Autodesk Inventor part; units mm, degrees
(part 2 of 2)
  spline S162 degree 2 poles (-0.0394, -200.6231) (-0.0431, -200.6898) (-0.0505, -200.8158) (-0.0505, -200.9121) knots 0 0 0 1 2 2 2
  spline S163 degree 2 poles (-0.0505, -200.9121) (-0.0505, -201.3864) (0.1348, -201.9681) (0.2755, -202.12) knots 0 0 0 1 2 2 2
  spline S164 degree 2 poles (0.2755, -202.12) (0.4052, -202.2645) (0.6868, -202.3793) (0.8461, -202.3793) knots 0 0 0 1 2 2 2
  spline S165 degree 2 poles (0.8461, -202.3793) (1.2166, -202.3793) (1.6723, -201.8532) (1.6723, -201.3271) knots 0 0 0 1 2 2 2
  line L137 (4.7364, -198.0074) -> (2.9469, -203.7761)
  line L138 (2.9469, -203.7761) -> (2.4282, -203.7761)
  line L139 (2.4282, -203.7761) -> (4.2103, -198.0074)
  line L140 (4.2103, -198.0074) -> (4.7364, -198.0074)
  line L141 (8.0598, -202.7832) -> (5.2403, -202.7832)
  line L142 (5.2403, -202.7832) -> (5.2403, -202.1348)
  spline S166 degree 2 poles (5.2403, -202.1348) (5.5441, -201.8495) (6.085, -201.3197) (6.3444, -201.0344) knots 0 0 0 1 2 2 2
  spline S167 degree 2 poles (6.3444, -201.0344) (6.8668, -200.4601) (7.2484, -199.771) (7.2484, -199.4042) knots 0 0 0 1 2 2 2
  spline S168 degree 2 poles (7.2484, -199.4042) (7.2484, -199.2115) (7.1298, -198.9225) (7.0224, -198.8299) knots 0 0 0 1 2 2 2
  spline S169 degree 2 poles (7.0224, -198.8299) (6.9149, -198.7373) (6.6334, -198.6447) (6.4629, -198.6447) knots 0 0 0 1 2 2 2
  spline S170 degree 2 poles (6.4629, -198.6447) (6.2999, -198.6447) (5.9665, -198.7262) (5.8146, -198.7892) knots 0 0 0 1 2 2 2
  spline S171 degree 2 poles (5.8146, -198.7892) (5.6849, -198.841) (5.4441, -198.9892) (5.37, -199.0411) knots 0 0 0 1 2 2 2
  line L143 (5.37, -199.0411) -> (5.3366, -199.0411)
  line L144 (5.3366, -199.0411) -> (5.3366, -198.389)
  spline S172 degree 2 poles (5.3366, -198.389) (5.5256, -198.2964) (6.2036, -198.1148) (6.5074, -198.1148) knots 0 0 0 1 2 2 2
  spline S173 degree 2 poles (6.5074, -198.1148) (7.1484, -198.1148) (7.8708, -198.7929) (7.8708, -199.3708) knots 0 0 0 1 2 2 2
  spline S174 degree 2 poles (7.8708, -199.3708) (7.8708, -199.6413) (7.7449, -200.0933) (7.6337, -200.286) knots 0 0 0 1 2 2 2
  spline S175 degree 2 poles (7.6337, -200.286) (7.5226, -200.4861) (7.2002, -200.8788) (7.0224, -201.0677) knots 0 0 0 1 2 2 2
  spline S176 degree 2 poles (7.0224, -201.0677) (6.7334, -201.3827) (6.0257, -202.057) (5.8146, -202.2534) knots 0 0 0 1 2 2 2
  line L145 (5.8146, -202.2534) -> (8.0598, -202.2534)
  line L146 (8.0598, -202.2534) -> (8.0598, -202.7832)
  spline S177 degree 2 poles (10.0531, -202.8869) (9.7122, -202.8869) (9.1528, -202.6831) (8.9564, -202.4942) knots 0 0 0 1 2 2 2
  spline S178 degree 2 poles (8.9564, -202.4942) (8.7638, -202.3089) (8.5637, -201.805) (8.5637, -201.5198) knots 0 0 0 1 2 2 2
  spline S179 degree 2 poles (8.5637, -201.5198) (8.5637, -201.1493) (8.9601, -200.5268) (9.338, -200.3416) knots 0 0 0 1 2 2 2
  line L147 (9.338, -200.3416) -> (9.338, -200.323)
  spline S180 degree 2 poles (9.338, -200.323) (9.0009, -200.1267) (8.6748, -199.6598) (8.6748, -199.3116) knots 0 0 0 1 2 2 2
  spline S181 degree 2 poles (8.6748, -199.3116) (8.6748, -198.7966) (9.4529, -198.1074) (10.0531, -198.1074) knots 0 0 0 1 2 2 2
  spline S182 degree 2 poles (10.0531, -198.1074) (10.6755, -198.1074) (11.4277, -198.7595) (11.4277, -199.2708) knots 0 0 0 1 2 2 2
  spline S183 degree 2 poles (11.4277, -199.2708) (11.4277, -199.5783) (11.0683, -200.1785) (10.7311, -200.349) knots 0 0 0 1 2 2 2
  line L148 (10.7311, -200.349) -> (10.7311, -200.3675)
  spline S184 degree 2 poles (10.7311, -200.3675) (11.1313, -200.5528) (11.5425, -201.0863) (11.5425, -201.5086) knots 0 0 0 1 2 2 2
  spline S185 degree 2 poles (11.5425, -201.5086) (11.5425, -202.094) (10.6904, -202.8869) (10.0531, -202.8869) knots 0 0 0 1 2 2 2
  spline S186 degree 2 poles (10.9127, -201.5679) (10.9127, -201.2863) (10.6904, -200.9529) (10.3754, -200.7825) knots 0 0 0 1 2 2 2
  spline S187 degree 2 poles (10.3754, -200.7825) (10.2717, -200.7232) (9.9234, -200.5861) (9.7048, -200.4972) knots 0 0 0 1 2 2 2
  spline S188 degree 2 poles (9.7048, -200.4972) (9.4529, -200.6639) (9.1824, -201.1604) (9.1824, -201.4753) knots 0 0 0 1 2 2 2
  spline S189 degree 2 poles (9.1824, -201.4753) (9.1824, -201.8903) (9.6826, -202.4312) (10.0605, -202.4312) knots 0 0 0 1 2 2 2
  spline S190 degree 2 poles (10.0605, -202.4312) (10.4458, -202.4312) (10.9127, -201.9681) (10.9127, -201.5679) knots 0 0 0 1 2 2 2
  spline S191 degree 2 poles (10.8275, -199.2782) (10.8275, -198.9707) (10.4162, -198.5594) (10.0494, -198.5594) knots 0 0 0 1 2 2 2
  spline S192 degree 2 poles (10.0494, -198.5594) (9.7159, -198.5594) (9.2899, -198.9262) (9.2899, -199.2412) knots 0 0 0 1 2 2 2
  spline S193 degree 2 poles (9.2899, -199.2412) (9.2899, -199.4672) (9.5085, -199.7821) (9.7271, -199.9081) knots 0 0 0 1 2 2 2
  spline S194 degree 2 poles (9.7271, -199.9081) (9.8197, -199.9599) (10.2124, -200.1415) (10.3717, -200.1934) knots 0 0 0 1 2 2 2
  spline S195 degree 2 poles (10.3717, -200.1934) (10.6385, -199.9896) (10.8275, -199.5561) (10.8275, -199.2782) knots 0 0 0 1 2 2 2
  line L149 (14.0027, -198.0074) -> (12.2131, -203.7761)
  line L150 (12.2131, -203.7761) -> (11.6944, -203.7761)
  line L151 (11.6944, -203.7761) -> (13.4765, -198.0074)
  line L152 (13.4765, -198.0074) -> (14.0027, -198.0074)
  line L153 (17.3261, -202.7832) -> (14.5065, -202.7832)
  line L154 (14.5065, -202.7832) -> (14.5065, -202.1348)
  spline S196 degree 2 poles (14.5065, -202.1348) (14.8104, -201.8495) (15.3513, -201.3197) (15.6106, -201.0344) knots 0 0 0 1 2 2 2
  spline S197 degree 2 poles (15.6106, -201.0344) (16.133, -200.4601) (16.5147, -199.771) (16.5147, -199.4042) knots 0 0 0 1 2 2 2
  spline S198 degree 2 poles (16.5147, -199.4042) (16.5147, -199.2115) (16.3961, -198.9225) (16.2887, -198.8299) knots 0 0 0 1 2 2 2
  spline S199 degree 2 poles (16.2887, -198.8299) (16.1812, -198.7373) (15.8996, -198.6447) (15.7292, -198.6447) knots 0 0 0 1 2 2 2
  spline S200 degree 2 poles (15.7292, -198.6447) (15.5662, -198.6447) (15.2327, -198.7262) (15.0808, -198.7892) knots 0 0 0 1 2 2 2
  spline S201 degree 2 poles (15.0808, -198.7892) (14.9511, -198.841) (14.7103, -198.9892) (14.6362, -199.0411) knots 0 0 0 1 2 2 2
  line L155 (14.6362, -199.0411) -> (14.6029, -199.0411)
  line L156 (14.6029, -199.0411) -> (14.6029, -198.389)
  spline S202 degree 2 poles (14.6029, -198.389) (14.7918, -198.2964) (15.4698, -198.1148) (15.7737, -198.1148) knots 0 0 0 1 2 2 2
  spline S203 degree 2 poles (15.7737, -198.1148) (16.4146, -198.1148) (17.1371, -198.7929) (17.1371, -199.3708) knots 0 0 0 1 2 2 2
  spline S204 degree 2 poles (17.1371, -199.3708) (17.1371, -199.6413) (17.0111, -200.0933) (16.9, -200.286) knots 0 0 0 1 2 2 2
  spline S205 degree 2 poles (16.9, -200.286) (16.7888, -200.4861) (16.4665, -200.8788) (16.2887, -201.0677) knots 0 0 0 1 2 2 2
  spline S206 degree 2 poles (16.2887, -201.0677) (15.9997, -201.3827) (15.292, -202.057) (15.0808, -202.2534) knots 0 0 0 1 2 2 2
  line L157 (15.0808, -202.2534) -> (17.3261, -202.2534)
  line L158 (17.3261, -202.2534) -> (17.3261, -202.7832)
  spline S207 degree 2 poles (20.7829, -200.4972) (20.7829, -201.7272) (20.0678, -202.8795) (19.3231, -202.8795) knots 0 0 0 1 2 2 2
  spline S208 degree 2 poles (19.3231, -202.8795) (18.5672, -202.8795) (17.8596, -201.705) (17.8596, -200.5009) knots 0 0 0 1 2 2 2
  spline S209 degree 2 poles (17.8596, -200.5009) (17.8596, -199.2634) (18.5747, -198.1185) (19.3231, -198.1185) knots 0 0 0 1 2 2 2
  spline S210 degree 2 poles (19.3231, -198.1185) (20.0752, -198.1185) (20.7829, -199.3042) (20.7829, -200.4972) knots 0 0 0 1 2 2 2
  spline S211 degree 2 poles (19.9974, -201.8903) (20.0863, -201.6643) (20.1604, -200.9677) (20.1604, -200.4972) knots 0 0 0 1 2 2 2
  spline S212 degree 2 poles (20.1604, -200.4972) (20.1604, -200.0266) (20.0863, -199.3338) (19.9937, -199.1004) knots 0 0 0 1 2 2 2
  spline S213 degree 2 poles (19.9937, -199.1004) (19.9011, -198.867) (19.5787, -198.6261) (19.3231, -198.6261) knots 0 0 0 1 2 2 2
  spline S214 degree 2 poles (19.3231, -198.6261) (19.0674, -198.6261) (18.7377, -198.867) (18.6413, -199.1078) knots 0 0 0 1 2 2 2
  spline S215 degree 2 poles (18.6413, -199.1078) (18.5487, -199.3412) (18.482, -200.0526) (18.482, -200.5009) knots 0 0 0 1 2 2 2
  spline S216 degree 2 poles (18.482, -200.5009) (18.482, -200.9825) (18.5413, -201.6272) (18.6376, -201.8791) knots 0 0 0 1 2 2 2
  spline S217 degree 2 poles (18.6376, -201.8791) (18.7266, -202.1163) (19.0563, -202.3719) (19.3231, -202.3719) knots 0 0 0 1 2 2 2
  spline S218 degree 2 poles (19.3231, -202.3719) (19.575, -202.3719) (19.9048, -202.1311) (19.9974, -201.8903) knots 0 0 0 1 2 2 2
  line L159 (24.1878, -202.7832) -> (21.3682, -202.7832)
  line L160 (21.3682, -202.7832) -> (21.3682, -202.1348)
  spline S219 degree 2 poles (21.3682, -202.1348) (21.6721, -201.8495) (22.213, -201.3197) (22.4723, -201.0344) knots 0 0 0 1 2 2 2
  spline S220 degree 2 poles (22.4723, -201.0344) (22.9948, -200.4601) (23.3764, -199.771) (23.3764, -199.4042) knots 0 0 0 1 2 2 2
  spline S221 degree 2 poles (23.3764, -199.4042) (23.3764, -199.2115) (23.2578, -198.9225) (23.1504, -198.8299) knots 0 0 0 1 2 2 2
  spline S222 degree 2 poles (23.1504, -198.8299) (23.0429, -198.7373) (22.7613, -198.6447) (22.5909, -198.6447) knots 0 0 0 1 2 2 2
  spline S223 degree 2 poles (22.5909, -198.6447) (22.4279, -198.6447) (22.0944, -198.7262) (21.9425, -198.7892) knots 0 0 0 1 2 2 2
  spline S224 degree 2 poles (21.9425, -198.7892) (21.8128, -198.841) (21.572, -198.9892) (21.4979, -199.0411) knots 0 0 0 1 2 2 2
  line L161 (21.4979, -199.0411) -> (21.4646, -199.0411)
  line L162 (21.4646, -199.0411) -> (21.4646, -198.389)
  spline S225 degree 2 poles (21.4646, -198.389) (21.6535, -198.2964) (22.3316, -198.1148) (22.6354, -198.1148) knots 0 0 0 1 2 2 2
  spline S226 degree 2 poles (22.6354, -198.1148) (23.2763, -198.1148) (23.9988, -198.7929) (23.9988, -199.3708) knots 0 0 0 1 2 2 2
  spline S227 degree 2 poles (23.9988, -199.3708) (23.9988, -199.6413) (23.8728, -200.0933) (23.7617, -200.286) knots 0 0 0 1 2 2 2
  spline S228 degree 2 poles (23.7617, -200.286) (23.6505, -200.4861) (23.3282, -200.8788) (23.1504, -201.0677) knots 0 0 0 1 2 2 2
  spline S229 degree 2 poles (23.1504, -201.0677) (22.8614, -201.3827) (22.1537, -202.057) (21.9425, -202.2534) knots 0 0 0 1 2 2 2
  line L163 (21.9425, -202.2534) -> (24.1878, -202.2534)
  line L164 (24.1878, -202.2534) -> (24.1878, -202.7832)
  spline S230 degree 2 poles (27.689, -201.3012) (27.689, -201.6531) (27.4556, -202.2497) (27.2592, -202.4497) knots 0 0 0 1 2 2 2
  spline S231 degree 2 poles (27.2592, -202.4497) (27.0555, -202.6609) (26.5442, -202.8795) (26.2366, -202.8795) knots 0 0 0 1 2 2 2
  spline S232 degree 2 poles (26.2366, -202.8795) (25.9291, -202.8795) (25.4215, -202.672) (25.2289, -202.4645) knots 0 0 0 1 2 2 2
  spline S233 degree 2 poles (25.2289, -202.4645) (24.9918, -202.2163) (24.725, -201.3827) (24.725, -200.7751) knots 0 0 0 1 2 2 2
  spline S234 degree 2 poles (24.725, -200.7751) (24.725, -200.1785) (24.9695, -199.2189) (25.2252, -198.8633) knots 0 0 0 1 2 2 2
  spline S235 degree 2 poles (25.2252, -198.8633) (25.4734, -198.515) (26.2589, -198.126) (26.7739, -198.126) knots 0 0 0 1 2 2 2
  spline S236 degree 2 poles (26.7739, -198.126) (26.9258, -198.126) (27.1925, -198.1556) (27.2926, -198.1889) knots 0 0 0 1 2 2 2
  line L165 (27.2926, -198.1889) -> (27.2926, -198.778)
  line L166 (27.2926, -198.778) -> (27.2666, -198.778)
  spline S237 degree 2 poles (27.2666, -198.778) (27.1814, -198.7336) (26.8702, -198.6558) (26.6924, -198.6558) knots 0 0 0 1 2 2 2
  spline S238 degree 2 poles (26.6924, -198.6558) (26.1218, -198.6558) (25.4215, -199.4264) (25.3549, -200.1822) knots 0 0 0 1 2 2 2
  spline S239 degree 2 poles (25.3549, -200.1822) (25.5734, -200.0303) (26.0329, -199.8636) (26.307, -199.8636) knots 0 0 0 1 2 2 2
  spline S240 degree 2 poles (26.307, -199.8636) (26.5738, -199.8636) (26.9739, -199.9711) (27.1925, -200.1341) knots 0 0 0 1 2 2 2
  spline S241 degree 2 poles (27.1925, -200.1341) (27.4445, -200.323) (27.689, -200.9084) (27.689, -201.3012) knots 0 0 0 1 2 2 2
  spline S242 degree 2 poles (27.0666, -201.3271) (27.0666, -201.0455) (26.9184, -200.6639) (26.7554, -200.5305) knots 0 0 0 1 2 2 2
  spline S243 degree 2 poles (26.7554, -200.5305) (26.6331, -200.4342) (26.3293, -200.3712) (26.17, -200.3712) knots 0 0 0 1 2 2 2
  spline S244 degree 2 poles (26.17, -200.3712) (25.9551, -200.3712) (25.5512, -200.5009) (25.3549, -200.6231) knots 0 0 0 1 2 2 2
  spline S245 degree 2 poles (25.3549, -200.6231) (25.3511, -200.6898) (25.3437, -200.8158) (25.3437, -200.9121) knots 0 0 0 1 2 2 2
  spline S246 degree 2 poles (25.3437, -200.9121) (25.3437, -201.3864) (25.529, -201.9681) (25.6698, -202.12) knots 0 0 0 1 2 2 2
  spline S247 degree 2 poles (25.6698, -202.12) (25.7995, -202.2645) (26.081, -202.3793) (26.2404, -202.3793) knots 0 0 0 1 2 2 2
  spline S248 degree 2 poles (26.2404, -202.3793) (26.6109, -202.3793) (27.0666, -201.8532) (27.0666, -201.3271) knots 0 0 0 1 2 2 2
  point P0 (0, 0)
  constraints: 2 other
emboss "Emboss1" sketch "Sketch14" operation cut depth 2.54 direction (-1, 0, 0)
sketch "Sketch16" plane through (5.08, 0, 0) normal (1, 0, 0) x (0, 0, -1)
  line L0 (-48.0867, -73.9362) -> (35.7333, -73.9362)
  line L1 (35.7333, -73.9362) -> (35.7333, -77.7462)
  line L2 (35.7333, -77.7462) -> (-48.0867, -77.7462)
  line L3 (-48.0867, -77.7462) -> (-48.0867, -73.9362)
  line L4 (36.3683, -211.0962) -> (-48.7217, -211.0962) projected
  line L5 (39.5433, 28.0448) -> (39.5433, -207.9212) projected
  line L6 (-51.8967, -207.9212) -> (-51.8967, 28.0448) projected
  point P0 (0, 0)
  point P1 (38.9083, -223.7962)
  point P2 (42.0833, -220.6212)
  point P3 (35.7333, -75.8412)
  point P4 (-48.0867, -75.8412)
  dimension "d195" = 3.81
  dimension "d692" = 137.16
  dimension "d796" = 3.81
  dimension "d797" = 3.81
  constraints: 8 end point, 2 midpoint, 2 parallel, 1 horizontal, 1 perpendicular, 2 other
  measures "d195" distance between parallel lines of L0 L2
  measures "d797" distance from line of L6 point (-48.087, -75.841)
extrude "Extrusion13" add sketch "Sketch16" along normal blind 5.08
sketch "Sketch17" plane through (24.13, 33.2264, 44.2767) normal (0, 1, 0) x (1, 0, 0)
  line L0 (-8.128, 57.15) -> (0, 57.15) projected
  line L1 (-0.0061, 57.15) -> (0.0392, 57.15)
  line L2 (0, 85.8266) -> (0, -9.6266) projected
  line L3 (0, 35.5801) -> (0, 35.5243)
  line L4 (5, -6.4516) -> (5, 82.6516) projected
  line L5 (0, 57.15) -> (5, 57.15)
  line L6 (5, 57.15) -> (5, 0)
  line L7 (5, 0) -> (0, 0)
  line L8 (0, 0) -> (0, 57.15)
  line L9 (0, 0) -> (-8.128, 0) projected
  point P0 (-24.13, 44.2767)
  point P1 (5, -23.8506)
  point P2 (5, 69.0626)
  point P3 (0, 0)
  point P4 (5, 57.15)
  point P5 (0, 57.15)
  point P6 (2.5, 0)
  point P7 (2.5, 57.15)
  dimension "d689" = 57.15
  dimension "d1196" = 0
  constraints: 12 end point, 4 point on line, 2 horizontal, 2 midpoint, 2 parallel, 1 perpendicular
  measures "d689" distance of point (2.5, 0) point (2.5, 57.15)
  measures "d1196" distance between parallel lines of L7 L9
extrude "Extrusion14" cut sketch "Sketch17" against normal blind 2.0066
sketch "Sketch18" plane through (0, 0, 0) normal (-1, 0, 0) x (0, 0, 1)
  arc A0 (52.5852, 32.6267) -> (53.9033, 29.2061) centre (54.6907, 31.4738) ccw projected
  circle A1 centre (54.6907, 31.4738) radius 4.5085
  arc A2 (-40.6969, 33.2264) -> (-41.5499, 29.2061) centre (-42.3373, 31.4738) ccw projected
  circle A3 centre (-42.3373, 31.4738) radius 4.5085
  arc A4 (-41.5499, -209.0826) -> (-40.2318, -212.5032) centre (-42.3373, -211.3502) ccw projected
  circle A5 centre (-42.3373, -211.3502) radius 4.5085
  arc A6 (52.5852, -212.5032) -> (53.9033, -209.0826) centre (54.6907, -211.3502) ccw projected
  circle A7 centre (54.6907, -211.3502) radius 4.5085
  point P0 (0, 0)
  point P1 (53.6972, 31.1766)
  point P2 (-40.9528, 32.4898)
  point P3 (-40.9528, 32.4898)
  point P4 (-41.3438, -211.0531)
  point P5 (53.6972, -211.0531)
  point P6 (-44.0899, -204.4909)
  point P7 (51.3633, -204.4909)
  point P8 (-41.0686, -213.1028)
  dimension "d209" = 9.017
  dimension "d210" = 9.017
  dimension "d211" = 9.017
  dimension "d212" = 9.017
  constraints: 4 centre point, 4 coincident
  measures "d209" diameter of A1
  measures "d210" diameter of A3
  measures "d211" diameter of A5
  measures "d212" diameter of A7
extrude "Extrusion15" [suppressed]
sketch "Sketch19" plane through (24.13, -51.5842, -41.5499) normal (0, 0, -1) x (-1, 0, 0)
  line L0 (7.62, 0) -> (0, 0) projected
  line L1 (-5, 79.629) -> (-5, -156.337) projected
  line L2 (0, 0) -> (-5, 0)
  line L3 (-5, 0) -> (-5, 12.7)
  line L4 (-5, 12.7) -> (0, 12.7)
  line L5 (0, 12.7) -> (0, 0)
  point P0 (24.13, 51.5842)
  point P1 (-5, -156.337)
  dimension "d216" = 5
  dimension "d219" = 12.7
  constraints: 8 end point, 2 parallel, 1 horizontal, 1 perpendicular, 1 point on line
  measures "d216" distance between parallel lines of L1 L5
  measures "d219" distance between parallel lines of L2 L4
extrude "Extrusion16" cut sketch "Sketch19" against normal blind 24.13
sketch "Sketch20" plane through (0, 0, 0) normal (-1, 0, 0) x (0, 0, 1)
  line L0 (-40.3379, 35.1568) -> (-38.2115, 31.4738)
  line L1 (-40.3379, 27.7908) -> (-38.2115, 31.4738)
  line L2 (-44.0209, 35.1568) -> (-40.3379, 35.1568)
  line L3 (-44.0209, 27.7908) -> (-40.3379, 27.7908)
  line L4 (-44.0209, 35.1568) -> (-46.1473, 31.4738)
  line L5 (-44.0209, 27.7908) -> (-46.1473, 31.4738)
  line L6 (56.6901, 35.1568) -> (58.8165, 31.4738)
  line L7 (56.6901, 27.7908) -> (58.8165, 31.4738)
  line L8 (53.0071, 35.1568) -> (56.6901, 35.1568)
  line L9 (53.0071, 27.7908) -> (56.6901, 27.7908)
  line L10 (53.0071, 35.1568) -> (50.8807, 31.4738)
  line L11 (53.0071, 27.7908) -> (50.8807, 31.4738)
  line L12 (50.7211, -60.3472) -> (52.8475, -64.0302)
  line L13 (50.7211, -67.7132) -> (52.8475, -64.0302)
  line L14 (47.0381, -60.3472) -> (50.7211, -60.3472)
  line L15 (47.0381, -67.7132) -> (50.7211, -67.7132)
  line L16 (47.0381, -60.3472) -> (44.9117, -64.0302)
  line L17 (47.0381, -67.7132) -> (44.9117, -64.0302)
  line L18 (-34.3689, -60.3472) -> (-32.2425, -64.0302)
  line L19 (-34.3689, -67.7132) -> (-32.2425, -64.0302)
  line L20 (-38.0519, -60.3472) -> (-34.3689, -60.3472)
  line L21 (-38.0519, -67.7132) -> (-34.3689, -67.7132)
  line L22 (-38.0519, -60.3472) -> (-40.1783, -64.0302)
  line L23 (-38.0519, -67.7132) -> (-40.1783, -64.0302)
  line L24 (-40.3379, -207.6672) -> (-38.2115, -211.3502)
  line L25 (-40.3379, -215.0332) -> (-38.2115, -211.3502)
  line L26 (-44.0209, -207.6672) -> (-40.3379, -207.6672)
  line L27 (-44.0209, -215.0332) -> (-40.3379, -215.0332)
  line L28 (-44.0209, -207.6672) -> (-46.1473, -211.3502)
  line L29 (-44.0209, -215.0332) -> (-46.1473, -211.3502)
  line L30 (56.6901, -207.6672) -> (58.8165, -211.3502)
  line L31 (56.6901, -215.0332) -> (58.8165, -211.3502)
  line L32 (53.0071, -207.6672) -> (56.6901, -207.6672)
  line L33 (53.0071, -215.0332) -> (56.6901, -215.0332)
  line L34 (53.0071, -207.6672) -> (50.8807, -211.3502)
  line L35 (53.0071, -215.0332) -> (50.8807, -211.3502)
  point P0 (0, 0)
  point P1 (-16.6833, 31.2198)
  point P2 (-42.1794, 27.7908)
  point P3 (54.8486, 27.7908)
  point P4 (54.6907, 31.4738)
  point P5 (48.8796, -67.7132)
  point P6 (-36.2104, -67.7132)
  point P7 (-42.1794, -215.0332)
  point P8 (54.8486, -215.0332)
  dimension "d1575" = 120
  dimension "d1576" = 120
  dimension "d1577" = 120
  dimension "d1578" = 120
  dimension "d1579" = 3.683
  dimension "d1580" = 3.683
  dimension "d1581" = 3.683
  dimension "d1582" = 3.683
  dimension "d1584" = 3.683
  dimension "d1586" = 3.683
  dimension "d1588" = 7.366
  dimension "d1589" = 7.9358
  dimension "d1592" = 7.9358
  dimension "d1593" = 0
  dimension "d1596" = 120
  dimension "d1597" = 120
  dimension "d1598" = 120
  dimension "d1599" = 120
  dimension "d1600" = 3.683
  dimension "d1601" = 3.683
  dimension "d1602" = 3.683
  dimension "d1603" = 3.683
  dimension "d1605" = 3.683
  dimension "d1607" = 3.683
  dimension "d1609" = 7.366
  dimension "d1610" = 7.9358
  dimension "d1613" = 7.9358
  dimension "d1614" = 0
  dimension "d1617" = 120
  dimension "d1618" = 120
  dimension "d1619" = 120
  dimension "d1620" = 120
  dimension "d1621" = 3.683
  dimension "d1622" = 3.683
  dimension "d1623" = 3.683
  dimension "d1624" = 3.683
  dimension "d1626" = 3.683
  dimension "d1628" = 3.683
  dimension "d1630" = 7.366
  dimension "d1631" = 7.9358
  dimension "d1634" = 7.9358
  dimension "d1635" = 0
  dimension "d1638" = 120
  dimension "d1639" = 120
  dimension "d1640" = 120
  dimension "d1641" = 120
  dimension "d1642" = 3.683
  dimension "d1643" = 3.683
  dimension "d1644" = 3.683
  dimension "d1645" = 3.683
  dimension "d1647" = 3.683
  dimension "d1649" = 3.683
  dimension "d1651" = 7.366
  dimension "d1652" = 7.9358
  dimension "d1655" = 7.9358
  dimension "d1656" = 0
  dimension "d1659" = 120
  dimension "d1660" = 120
  dimension "d1661" = 120
  dimension "d1662" = 120
  dimension "d1663" = 3.683
  dimension "d1664" = 3.683
  dimension "d1665" = 3.683
  dimension "d1666" = 3.683
  constraints: 72 end point, 12 horizontal, 6 midpoint
  measures "d1575" angle of L3 L5
  measures "d1576" angle of L2 L4
  measures "d1577" angle of L1 L3
  measures "d1578" angle of L0 L2
  measures "d1579" distance of L5.start L3.end
  measures "d1580" distance of L4.start L2.end
  measures "d1581" vertical distance of L3.end L1.end
  measures "d1582" vertical distance of L4.end L4.start
  measures "d1584" vertical distance of L5.end L5.start
  measures "d1586" vertical distance of L0.end L2.end
  measures "d1588" distance of L3.end L2.end
  measures "d1589" distance of L4.end L0.end
  measures "d1592" distance of L1.end L5.end
  measures "d1593" distance of L4.end L5.end
  measures "d1596" angle of L9 L11
  measures "d1597" angle of L8 L10
  measures "d1598" angle of L7 L9
  measures "d1599" angle of L6 L8
  measures "d1600" distance of L11.start L9.end
  measures "d1601" distance of L10.start L8.end
  measures "d1602" vertical distance of L9.end L7.end
  measures "d1603" vertical distance of L10.end L10.start
  measures "d1605" vertical distance of L11.end L11.start
  measures "d1607" vertical distance of L6.end L8.end
  measures "d1609" distance of L9.end L8.end
  measures "d1610" distance of L10.end L6.end
  measures "d1613" distance of L7.end L11.end
  measures "d1614" distance of L10.end L11.end
  measures "d1617" angle of L15 L17
  measures "d1618" angle of L14 L16
  measures "d1619" angle of L13 L15
  measures "d1620" angle of L12 L14
  measures "d1621" distance of L15.start L15.end
  measures "d1622" distance of L14.start L14.end
  measures "d1623" vertical distance of L15.end L13.end
  measures "d1624" vertical distance of L16.end L14.start
  measures "d1626" vertical distance of L17.end L15.start
  measures "d1628" vertical distance of L12.end L14.end
  measures "d1630" distance of L15.end L14.end
  measures "d1631" distance of L16.end L12.end
  measures "d1634" distance of L13.end L17.end
  measures "d1635" distance of L16.end L17.end
  measures "d1638" angle of L21 L23
  measures "d1639" angle of L20 L22
  measures "d1640" angle of L19 L21
  measures "d1641" angle of L18 L20
  measures "d1642" distance of L21.start L21.end
  measures "d1643" distance of L20.start L20.end
  measures "d1644" vertical distance of L21.end L19.end
  measures "d1645" vertical distance of L22.end L20.start
  measures "d1647" vertical distance of L23.end L21.start
  measures "d1649" vertical distance of L18.end L20.end
  measures "d1651" distance of L21.end L20.end
  measures "d1652" distance of L22.end L18.end
  measures "d1655" distance of L19.end L23.end
  measures "d1656" distance of L22.end L23.end
  measures "d1659" angle of L27 L29
  measures "d1660" angle of L26 L28
  measures "d1661" angle of L25 L27
  measures "d1662" angle of L24 L26
  measures "d1663" distance of L27.start L27.end
  measures "d1664" distance of L26.start L26.end
  measures "d1665" vertical distance of L27.end L25.end
  measures "d1666" vertical distance of L28.end L26.start
extrude "Extrusion18" cut sketch "Sketch20" against normal blind 4
sketch "Sketch21" plane through (5.08, 0, 0) normal (1, 0, 0) x (0, 0, -1)
  line L0 (-51.8967, -207.9212) -> (-51.8967, 28.0448) projected
  line L1 (42.0833, -69.6717) -> (42.0833, -83.8957)
  line L2 (41.5499, -209.9278) -> (41.5499, -51.5842) projected
  line L3 (-51.8967, -83.8422) -> (-51.8967, -69.6182)
  line L4 (-45.0387, -58.8939) -> (-45.0387, -69.23)
  line L5 (-46.7701, -72.0578) -> (-49.9197, -73.6657)
  line L6 (-51.2708, -74.9867) -> (-51.8967, -76.1476)
  line L7 (-46.7701, -56.0661) -> (-49.9197, -54.4582)
  line L8 (-51.3039, -53.074) -> (-51.8967, -51.9128)
  arc A0 (-49.9197, -73.6657) -> (-51.2708, -74.9867) centre (-48.4761, -76.4935) ccw
  arc A1 (-46.7701, -72.0578) -> (-45.0387, -69.23) centre (-48.2137, -69.23) ccw
  arc A2 (-45.0387, -58.8939) -> (-46.7701, -56.0661) centre (-48.2137, -58.8939) ccw
  arc A3 (-51.3039, -53.074) -> (-49.9197, -54.4582) centre (-48.4761, -51.6304) ccw
  line L9 (-51.8967, -51.9128) -> (-51.8967, -76.1476)
  line L10 (32.6853, -69.1835) -> (32.6853, -58.8478)
  line L11 (34.4169, -56.0198) -> (37.5665, -54.4123)
  line L12 (38.9275, -53.0729) -> (39.5433, -51.9128)
  line L13 (34.4169, -72.0115) -> (37.5665, -73.619)
  line L14 (38.9275, -74.9584) -> (39.5433, -76.1184)
  arc A4 (38.9275, -74.9584) -> (37.5665, -73.619) centre (36.1231, -76.447) ccw
  arc A5 (32.6853, -69.1835) -> (34.4169, -72.0115) centre (35.8603, -69.1835) ccw
  arc A6 (37.5665, -54.4123) -> (38.9275, -53.0729) centre (36.1231, -51.5843) ccw
  arc A7 (34.4169, -56.0198) -> (32.6853, -58.8478) centre (35.8603, -58.8478) ccw
  line L15 (39.5433, -51.9128) -> (39.5433, -76.1184)
  line L16 (39.5433, -51.9128) -> (39.5433, -76.1184)
  circle A8 centre (36.3683, -64.0302) radius 2.4005 projected
  line L17 (39.5433, -51.5842) -> (39.5433, -38.8842) projected
  circle A9 centre (36.3683, -64.0302) radius 2.4005
  circle A10 centre (-48.7217, -64.0302) radius 2.4005 projected
  circle A11 centre (-48.7217, -64.0302) radius 2.4005
  point P0 (0, 0)
  point P1 (-43.0067, -58.9502)
  point P2 (-50.8011, -74.1156)
  point P3 (-50.8361, -53.9904)
  point P4 (-43.0067, -74.3297)
  point P5 (-40.8318, -77.7462)
  point P6 (-51.1222, -64.0302)
  point P7 (-51.1222, -64.0302)
  point P8 (-51.1222, -64.0302)
  point P9 (-51.1222, -64.0302)
  point P10 (38.4582, -53.9572)
  point P11 (42.0833, -76.1184)
  point P12 (35.8863, -63.7762)
  point P13 (38.2733, -66.4307)
  point P14 (39.5433, -61.7153)
  point P15 (39.5433, -66.3452)
  point P16 (-51.8967, -66.3452)
  point P17 (-51.8967, -61.7153)
  dimension "d785" = 6.858
  dimension "d786" = 117.044
  dimension "d787" = 117.044
  dimension "d792" = 2.032
  dimension "d793" = 3.175
  dimension "d794" = 3.1496
  dimension "d795" = 3.1496
  dimension "d917" = 24.2348
  dimension "d1144" = 145
  dimension "d1145" = 145
  dimension "d1146" = 117.04
  dimension "d1147" = 117.04
  dimension "d1148" = 3.175
  dimension "d1149" = 3.175
  dimension "d1150" = 3.1496
  dimension "d1151" = 2.0443
  dimension "d1152" = 3.1496
  dimension "d1153" = 24.2056
  dimension "d1155" = 0
  dimension "d1159" = 12.1174
  dimension "d1198" = 12.1174
  constraints: 30 end point, 16 point on circle, 16 tangent, 10 centre point, 9 point on line, 5 equal radius, 2 coincident, 2 vertical, 1 collinear, 1 parallel, 1 perpendicular, 4 other
  measures "d785" distance between parallel lines of L0 L4
  measures "d786" angle of L5 L4
  measures "d787" angle of L7 L4
  measures "d792" vertical distance of point (-50.801, -74.116) L6.end
  measures "d793" radius of A0
  measures "d794" horizontal distance of L5.start L5.end
  measures "d795" horizontal distance of L7.start L7.end
  measures "d917" distance of L6.end L8.end
  measures "d1144" angle of L11 L12
  measures "d1145" angle of L14 L13
  measures "d1146" angle of L13 L10
  measures "d1147" angle of L10 L11
  measures "d1148" radius of A4
  measures "d1149" radius of A6
  measures "d1150" horizontal distance of L11.start L11.end
  measures "d1151" vertical distance of L12.end point (38.458, -53.957)
  measures "d1152" horizontal distance of L13.start L13.end
  measures "d1153" distance of L14.end L12.end
  measures "d1155" distance between parallel lines of L17 L15
  measures "d1159" vertical distance of point (36.368, -64.03) L12.end
  measures "d1198" vertical distance of point (-48.722, -64.03) L8.end
extrude "Extrusion19" add sketch "Sketch21" along normal blind 24.13
sketch "Sketch22" plane through (16.08, -230.1462, -3.2973) normal (0, -1, 0) x (1, 0, 0)
  circle A0 centre (2.2292, -12.1283) radius 2.032
  line L0 (-16.08, -45.136) -> (8.05, -45.136) projected
  circle A1 centre (10.002, -12.1283) radius 2.032
  line L1 (13.05, 48.9456) -> (13.05, -37.6176) projected
  point P0 (-16.08, 3.2973)
  dimension "d445" = 4.064
  dimension "d446" = 33.0076
  dimension "d449" = 4.064
  dimension "d450" = 3.048
  constraints: 2 centre point
  measures "d445" diameter of A0
  measures "d446" distance from line of L0 A0.centre
  measures "d449" diameter of A1
  measures "d450" distance from line of L1 A1.centre
extrude "Extrusion20" [suppressed]
fillet "Fillet6" radius 0.508 2 edges at (16.002, 37.5698, 15.7017) (20.066, 37.5698, -12.8733)
sketch "Sketch23" plane through (22.86, -225.8028, -3.2973) normal (0, -1, 0) x (1, 0, 0)
  line L0 (1.27, -37.6176) -> (1.27, 48.9456) projected
  line L1 (6.27, 48.9456) -> (6.27, -37.6176) projected
  line L2 (0, 10) -> (6.27, 10)
  line L3 (6.27, 10) -> (6.27, -0.0129)
  line L4 (6.27, -0.0129) -> (0, -0.0129)
  line L5 (0, -0.0129) -> (0, 10)
  point P0 (-22.86, 3.2973)
  point P1 (1.27, 48.9456)
  constraints: 8 end point, 2 parallel, 1 horizontal, 1 perpendicular, 1 point on line, 1 other
extrude "Extrusion21" [suppressed]
sketch "Sketch24" plane through (8.636, -223.7962, -3.2973) normal (0, 1, 0) x (1, 0, 0)
  circle A0 centre (9.652, -31.318) radius 4.445
  line L0 (-3.556, 35.611) -> (-3.556, -46.939) projected
  point P0 (-8.636, -3.2973)
  point P1 (15.494, -56.464)
  dimension "d673" = 25.146
  dimension "d674" = 13.208
  dimension "d677" = 8.89
  constraints: 1 centre point
  measures "d673" vertical distance of point (15.494, -56.464) A0.centre
  measures "d674" distance from line of L0 A0.centre
  measures "d677" diameter of A0
extrude "Extrusion22" [suppressed]
sketch "Sketch25" plane through (5.08, 0, 0) normal (1, 0, 0) x (0, 0, -1)
  line L0 (-51.8967, 15.9798) -> (20.6609, 15.9798)
  line L1 (10.5009, 3.2798) -> (-51.8967, 3.2798)
  line L2 (-51.8967, 3.2798) -> (-51.8967, 15.9798)
  circle A0 centre (-34.1167, 9.6298) radius 2.4005 projected
  circle A1 centre (2.8809, 9.6298) radius 2.4005 projected
  circle A2 centre (-15.6179, 9.6298) radius 2.4005 projected
  line L3 (-51.8967, -207.9212) -> (-51.8967, 28.0448) projected
  line L4 (39.5433, 28.0448) -> (39.5433, -38.8842) projected
  line L5 (20.6609, 15.9798) -> (39.5433, 15.9798)
  line L6 (39.5433, 15.9798) -> (39.5433, 3.2798)
  line L7 (39.5433, 3.2798) -> (10.5009, 3.2798)
  point P0 (0, 0)
  point P1 (-15.6179, 15.9798)
  point P2 (-46.8167, -36.8286)
  point P3 (-51.8967, 28.0448)
  point P4 (42.0833, -36.6918)
  point P5 (39.5433, -38.8842)
  point P6 (-51.8967, -207.9212)
  dimension "d680" = 6.35
  dimension "d681" = 6.35
  dimension "d682" = 0
  dimension "d685" = 0
  dimension "d686" = 12.7
  constraints: 12 end point, 2 horizontal, 2 parallel, 1 midpoint, 1 perpendicular, 2 other
  measures "d680" distance of point (-15.618, 15.98) A2.centre
  measures "d681" distance from line of L1 A2.centre
  measures "d682" horizontal extent of L2
  measures "d685" horizontal extent of L6
  measures "d686" distance between parallel lines of L7 L5
extrude "Extrusion23" add sketch "Sketch25" along normal blind 10.16
sketch "Sketch26" plane through (0, -217.4462, -45.2583) normal (0, -1, 0) x (1, 0, 0)
  line L0 (29.13, 93.345) -> (10.3097, 93.345)
  line L1 (10.3097, 9.525) -> (29.13, 9.525)
  line L2 (29.13, 9.525) -> (29.13, 93.345)
  line L3 (0, -3.175) -> (24.13, -3.175) projected
  line L4 (24.13, 106.045) -> (0, 106.045) projected
  line L5 (29.13, 95.9866) -> (29.13, 6.8834) projected
  line L6 (8.7811, 93.345) -> (8.7811, 85.0428)
  line L7 (10.3097, 93.345) -> (8.7811, 93.345)
  line L8 (8.7811, 93.345) -> (8.7811, 9.525)
  line L9 (10.3097, 9.525) -> (8.7811, 9.525)
  point P0 (0, 45.2583)
  point P1 (29.13, 51.961)
  dimension "d832" = 12.7
  dimension "d833" = 12.7
  dimension "d837" = 0
  constraints: 14 end point, 2 horizontal, 2 perpendicular, 1 parallel, 1 vertical
  measures "d832" distance between parallel lines of L3 L1
  measures "d833" distance between parallel lines of L4 L0
  measures "d837" distance between parallel lines of L5 L2
extrude "Extrusion24" cut sketch "Sketch26" against normal blind 7.62
fillet "Fillet7" radius 0.762 4 edges at (17.2199, -217.4462, 48.0867) (9.5454, -217.4462, 48.0867) (17.2199, -217.4462, -35.7333) (9.5454, -217.4462, -35.7333)
sketch "Sketch27" plane through (0, -214.2712, -48.4333) normal (0, 0, -1) x (-1, 0, 0)
  line L0 (-29.13, 243.4773) -> (-29.13, 5.1887) projected
  line L1 (-29.13, 161.6205) -> (-16.51, 161.6205)
  line L2 (-16.51, 161.6205) -> (-16.51, 162.687)
  line L3 (-16.51, 162.687) -> (-29.13, 162.687)
  line L4 (-29.21, 138.1528) -> (-29.21, 162.3584) projected
  line L5 (-29.13, 161.6205) -> (-29.21, 161.6205)
  line L6 (-29.21, 161.6205) -> (-29.21, 162.687)
  line L7 (-29.21, 162.687) -> (-29.13, 162.687)
  line L8 (-16.51, 175.387) -> (-16.51, 162.687) projected
  point P0 (0, 214.2712)
  dimension "d1705" = 0.08
  dimension "d1706" = 0
  constraints: 12 end point, 2 horizontal, 2 parallel, 2 perpendicular, 2 point on line
  measures "d1705" distance between parallel lines of L4 L0
  measures "d1706" distance between parallel lines of L8 L2
extrude "Extrusion25" cut sketch "Sketch27" against normal blind 25.4
fillet "Fillet8" radius 0.508 4 edges at (20.32, -38.8842, -48.4333) (16.51, -45.2342, -48.4333) (16.51, -52.1175, -48.4333) (20.32, -52.6507, -48.4333)
body "Solid1"
